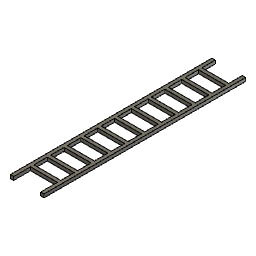
FuelTankLadder (Autodesk Fusion 360 design; units mm, degrees)
Autodesk Fusion 360 part; units mm, degrees
sketch "Sketch1" plane through (0, 0, 0) normal (0, 1, 0) x (1, 0, 0)
  line L0 (0, 0) -> (0.5, 0)
  line L1 (0.5, 0) -> (0.5, 30)
  line L2 (0.5, 30) -> (0, 30)
  line L3 (0, 30) -> (0, 0)
  line L4 (4.5, 0) -> (5, 0)
  line L5 (5, 0) -> (5, 30)
  line L6 (5, 30) -> (4.5, 30)
  line L7 (4.5, 30) -> (4.5, 0)
  line L8 (0.5, 2.5) -> (4.5, 2.5)
  line L9 (4.5, 2.5) -> (4.5, 3)
  line L10 (4.5, 3) -> (0.5, 3)
  line L11 (0.5, 3) -> (0.5, 2.5)
  line L12 (0.5, 5) -> (4.5, 5)
  line L13 (4.5, 5) -> (4.5, 5.5)
  line L14 (4.5, 5.5) -> (0.5, 5.5)
  line L15 (0.5, 5.5) -> (0.5, 5)
  line L16 (0.5, 7.5) -> (4.5, 7.5)
  line L17 (4.5, 7.5) -> (4.5, 8)
  line L18 (4.5, 8) -> (0.5, 8)
  line L19 (0.5, 8) -> (0.5, 7.5)
  line L20 (0.5, 10) -> (4.5, 10)
  line L21 (4.5, 10) -> (4.5, 10.5)
  line L22 (4.5, 10.5) -> (0.5, 10.5)
  line L23 (0.5, 10.5) -> (0.5, 10)
  line L24 (0.5, 12.5) -> (4.5, 12.5)
  line L25 (4.5, 12.5) -> (4.5, 13)
  line L26 (4.5, 13) -> (0.5, 13)
  line L27 (0.5, 13) -> (0.5, 12.5)
  line L28 (0.5, 15) -> (4.5, 15)
  line L29 (4.5, 15) -> (4.5, 15.5)
  line L30 (4.5, 15.5) -> (0.5, 15.5)
  line L31 (0.5, 15.5) -> (0.5, 15)
  line L32 (0.5, 17.5) -> (4.5, 17.5)
  line L33 (4.5, 17.5) -> (4.5, 18)
  line L34 (4.5, 18) -> (0.5, 18)
  line L35 (0.5, 18) -> (0.5, 17.5)
  line L36 (0.5, 20) -> (4.5, 20)
  line L37 (4.5, 20) -> (4.5, 20.5)
  line L38 (4.5, 20.5) -> (0.5, 20.5)
  line L39 (0.5, 20.5) -> (0.5, 20)
  line L40 (0.5, 22.5) -> (4.5, 22.5)
  line L41 (4.5, 22.5) -> (4.5, 23)
  line L42 (4.5, 23) -> (0.5, 23)
  line L43 (0.5, 23) -> (0.5, 22.5)
  line L44 (0.5, 25) -> (4.5, 25)
  line L45 (4.5, 25) -> (4.5, 25.5)
  line L46 (4.5, 25.5) -> (0.5, 25.5)
  line L47 (0.5, 25.5) -> (0.5, 25)
  line L48 (0.5, 27.5) -> (4.5, 27.5)
  line L49 (4.5, 27.5) -> (4.5, 28)
  line L50 (4.5, 28) -> (0.5, 28)
  line L51 (0.5, 28) -> (0.5, 27.5)
  dimension "d1" = 0.5
  dimension "d2" = 30
  dimension "d3" = 0.5
  dimension "d4" = 5
  dimension "d5" = 4
  dimension "d6" = 0.5
  dimension "d7" = 0.5
  dimension "d8" = 2
  dimension "d9" = 0.5
  dimension "d10" = 2
  dimension "d11" = 0.5
  dimension "d12" = 2
  dimension "d13" = 0.5
  dimension "d14" = 2
  dimension "d15" = 0.5
  dimension "d16" = 2
  dimension "d17" = 0.5
  dimension "d18" = 2
  dimension "d19" = 0.5
  dimension "d20" = 2
  dimension "d21" = 0.5
  dimension "d22" = 2
  dimension "d23" = 0.5
  dimension "d24" = 2
  dimension "d25" = 0.5
  dimension "d26" = 2
  constraint horizontal L0
  constraint vertical L1
  constraint horizontal L2
  constraint vertical L3
  constraint coincident L0.start L3.end
  constraint horizontal L4
  constraint vertical L5
  constraint horizontal L6
  constraint vertical L7
  constraint horizontal L8
  constraint vertical L9
  constraint horizontal L10
  constraint vertical L11
  constraint coincident L1 L8.start
  constraint horizontal L12
  constraint vertical L13
  constraint horizontal L14
  constraint vertical L15
  constraint coincident L1 L12.start
  constraint horizontal L16
  constraint vertical L17
  constraint horizontal L18
  constraint vertical L19
  constraint coincident L1 L16.start
  constraint horizontal L20
  constraint vertical L21
  constraint horizontal L22
  constraint vertical L23
  constraint coincident L1 L20.start
  constraint horizontal L24
  constraint vertical L25
  constraint horizontal L26
  constraint vertical L27
  constraint coincident L1 L24.start
  constraint horizontal L28
  constraint vertical L29
  constraint horizontal L30
  constraint vertical L31
  constraint midpoint L1 L28.start
  constraint horizontal L32
  constraint vertical L33
  constraint horizontal L34
  constraint vertical L35
  constraint coincident L7 L33.end
  constraint coincident L1 L32.start
  constraint horizontal L36
  constraint vertical L37
  constraint horizontal L38
  constraint vertical L39
  constraint coincident L1 L36.start
  constraint horizontal L40
  constraint vertical L41
  constraint horizontal L42
  constraint vertical L43
  constraint coincident L1 L40.start
  constraint horizontal L44
  constraint vertical L45
  constraint horizontal L46
  constraint vertical L47
  constraint coincident L1 L44.start
  constraint horizontal L48
  constraint vertical L49
  constraint horizontal L50
  constraint vertical L51
  constraint coincident L1 L48.start
  measures "d1" distance of L0.start L0.end
  measures "d2" distance of L0.start L2.end
  measures "d3" distance of L4.start L4.end
  measures "d4" distance of L2.end L5.end
  measures "d5" distance of L8.start L8.end
  measures "d6" distance of L8.start L10.end
  measures "d7" distance of L12.start L14.end
  measures "d8" distance of L10 L12
  measures "d9" distance of L16.start L18.end
  measures "d10" distance of L14 L16
  measures "d11" distance of L20.start L22.end
  measures "d12" distance of L18 L20
  measures "d13" distance of L24.start L26.end
  measures "d14" distance of L22 L24
  measures "d15" distance of L28.start L30.end
  measures "d16" distance of L26 L28
  measures "d17" distance of L32.start L34.end
  measures "d18" distance of L30 L32
  measures "d19" distance of L36.start L38.end
  measures "d20" distance of L34 L36
  measures "d21" distance of L40.start L42.end
  measures "d22" distance of L38 L40
  measures "d23" distance of L44.start L46.end
  measures "d24" distance of L42 L44
  measures "d25" distance of L48.start L50.end
  measures "d26" distance of L46 L48
extrude "Extrude1" add sketch "Sketch1" along normal blind 0.5 contours L0 L1 L2 L3 L11 L15 L19 L23 L27 L31 L35 L39 L43 L47 L51 | L1 L7 L8 L9 L10 L11 | L4 L5 L6 L7 L9 L13 L17 L21 L25 L29 L33 L37 L41 L45 L49 | L1 L7 L48 L49 L50 L51 | L1 L7 L12 L13 L14 L15 | L1 L7 L44 L45 L46 L47 | L1 L7 L16 L17 L18 L19 | L1 L7 L40 L41 L42 L43 | L1 L7 L20 L21 L22 L23 | L1 L7 L36 L37 L38 L39 | L1 L7 L24 L25 L26 L27 | L1 L7 L32 L33 L34 L35 | L1 L7 L28 L29 L30 L31
